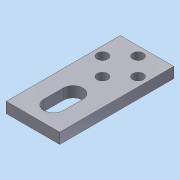
# Autodesk Inventor part: Micro Limit Switch Plate
Saved by Autodesk Inventor 2013 (Build 170138000, 138)
## iProperties
Created: 2013-12-08
Part Number: Micro Limit Switch Plate
Material: Aluminum 6061
Document SubType Name: Modeling
Designer: Jon Hollander
Density: 2.71 g/cm^3
Catalog Web Link: www.openbuildspartstore.com
Vendor: OpenBuilds
Mass: 3.23344 g
Surface Area: 12.7537 cm^2
Volume: 1.19315 cm^3
Author: Work
Autodesk Inventor part; units mm, degrees
ref_plane "YZ Plane" through (0, 0, 0) normal (1, 0, 0) x (0, 1, 0)
ref_plane "XZ Plane" through (0, 0, 0) normal (0, 1, 0) x (-1, 0, 0)
ref_plane "XY Plane" through (0, 0, 0) normal (0, 0, 1) x (1, 0, 0)
sketch "Sketch1" plane through (0, 0, 0) normal (0, 0, 1) x (1, 0, 0)
  line L0 (-7.5, 16) -> (7.5, 16)
  line L1 (7.5, 16) -> (7.5, -16)
  line L2 (7.5, -16) -> (-7.5, -16)
  line L3 (-7.5, -16) -> (-7.5, 16)
  line L4 (-7.5, 16) -> (7.5, -16) construction
  line L5 (7.5, 16) -> (-7.5, -16) construction
  point P0 (0, 0)
  dimension "d0" = 32
  dimension "d2" = 15
  constraints: 12 end point, 2 midpoint, 2 parallel, 1 horizontal, 1 perpendicular
  measures "d0" distance of L2.end L0.start
  measures "d2" distance of L1.end L2.end
extrude "Extrusion1" add sketch "Sketch1" along normal mid plane 3
sketch "Sketch2" plane through (0, 0, 1.5) normal (0, 0, 1) x (1, 0, 0)
  line L0 (7.5, 16) -> (-7.5, 16) projected
  line L1 (-7.5, -16) -> (7.5, -16) projected
  line L2 (0, 16) -> (0, -16) construction
  point P0 (0, 0)
  point P1 (0, 13.5)
  point P2 (0, 3.5)
  point P3 (-5, 8.5)
  point P4 (5, 8.5)
  dimension "d5" = 10
  dimension "d7" = 10
  dimension "d8" = 5
  dimension "d9" = 2.5
  dimension "d10" = 5
  constraints: 2 end point, 2 midpoint, 1 horizontal alignment, 1 point on line, 1 vertical alignment
  measures "d5" distance of point (0, 3.5) point (0, 13.5)
  measures "d7" distance of point (5, 8.5) point (-5, 8.5)
  measures "d8" distance from line of L2 point (5, 8.5)
  measures "d9" distance from line of L0 point (0, 13.5)
  measures "d10" horizontal distance of point (0, 13.5) point (5, 8.5)
hole "Hole1" at (0, 13.5, 1.5) at (0, 3.5, 1.5) at (-5, 8.5, 1.5) at (5, 8.5, 1.5) direction (0, 0, -1) diameter 3 end through all
sketch "Sketch3" plane through (0, 0, 1.5) normal (0, 0, 1) x (1, 0, 0)
  line L0 (-7.5, -16) -> (7.5, -16) projected
  line L1 (7.5, -16) -> (7.5, 16) projected
  line L2 (0, -23.093) -> (0, 0) construction
  line L3 (-2.75, -4.73) -> (2.75, -4.73)
  line L4 (2.75, -4.73) -> (2.75, -10.23)
  line L5 (2.75, -10.23) -> (-2.75, -10.23)
  line L6 (-2.75, -10.23) -> (-2.75, -4.73)
  line L7 (-2.75, -4.73) -> (2.75, -10.23) construction
  line L8 (2.75, -4.73) -> (-2.75, -10.23) construction
  arc A0 (-2.75, -10.23) -> (2.75, -10.23) centre (0, -10.23) ccw
  arc A1 (2.75, -4.73) -> (-2.75, -4.73) centre (0, -4.73) ccw
  point P0 (0, -7.48)
  dimension "d18" = 5.5
  dimension "d20" = 5.5
  dimension "d21" = 3.02
  constraints: 14 end point, 4 midpoint, 4 point on circle, 3 parallel, 2 centre point, 1 horizontal, 1 perpendicular, 1 point on line
  measures "d18" distance of L4.end L5.end
  measures "d20" distance between parallel lines of L3 L5
  measures "d21" distance edge to line of A0 L0
extrude "Extrusion2" cut sketch "Sketch3" against normal through all
body "Solid1"
